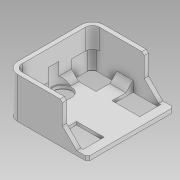
# Autodesk Inventor part: StandardPillarCover
Saved by Autodesk Inventor 2021 (Build 250183000, 183)
## iProperties
Created: 2021-03-17
Part Number: StandardPillarCover
Material: 一般
Document SubType Name: Modeling
Designer: kumagai
Density: 1 g/cm^3
Appearance: 既定
Author: kumagai
Autodesk Inventor part; units mm, degrees
ref_plane "YZ Plane" through (0, 0, 0) normal (1, 0, 0) x (0, 1, 0)
ref_plane "XZ Plane" through (0, 0, 0) normal (0, 1, 0) x (-1, 0, 0)
ref_plane "XY Plane" through (0, 0, 0) normal (0, 0, 1) x (1, 0, 0)
sketch "スケッチ1" plane through (0, 0, 0) normal (0, 1, 0) x (-1, 0, 0)
  line L0 (0, -22.1598) -> (0, 22.1598) projected
  line L1 (-9.6657, 0) -> (57.9941, 0) projected
  line L2 (43.5, -15) -> (19.2, -15)
  line L3 (19.2, -15) -> (19.2, 15)
  line L4 (19.2, 15) -> (43.5, 15)
  line L5 (47.5, 11) -> (47.5, -11)
  arc A0 (43.5, -15) -> (47.5, -11) centre (43.5, -11) ccw
  arc A1 (47.5, 11) -> (43.5, 15) centre (43.5, 11) ccw
  line L6 (44.65, -13.5) -> (37.45, -13.5)
  line L7 (37.45, -13.5) -> (37.45, -6.2)
  line L8 (37.45, -6.2) -> (46.15, -6.2)
  line L9 (46.15, -6.2) -> (46.15, -12)
  line L10 (31.85, -13.5) -> (22.25, -13.5)
  line L11 (22.25, -13.5) -> (22.25, -6.2)
  line L12 (22.25, -6.2) -> (31.85, -6.2)
  line L13 (31.85, -6.2) -> (31.85, -13.5)
  line L14 (22.25, 6.2) -> (31.85, 6.2)
  line L15 (31.85, 6.2) -> (31.85, 13.5)
  line L16 (31.85, 13.5) -> (22.25, 13.5)
  line L17 (22.25, 13.5) -> (22.25, 6.2)
  line L18 (37.45, 6.2) -> (46.15, 6.2)
  line L19 (46.15, 6.2) -> (46.15, 12)
  line L20 (44.65, 13.5) -> (37.45, 13.5)
  line L21 (37.45, 13.5) -> (37.45, 6.2)
  arc A2 (44.65, -13.5) -> (46.15, -12) centre (44.65, -12) ccw
  arc A3 (46.15, 12) -> (44.65, 13.5) centre (44.65, 12) ccw
  line L22 (28, -13.5) -> (43.5, -13.5)
  line L23 (46, -11) -> (46, 11)
  line L24 (43.5, 13.5) -> (28, 13.5)
  arc A4 (43.5, -13.5) -> (46, -11) centre (43.5, -11) ccw
  arc A5 (46, 11) -> (43.5, 13.5) centre (43.5, 11) ccw
  circle A6 centre (43, 0) radius 3.2
  line L25 (28, -13.5) -> (28, -15)
  line L26 (28, 13.5) -> (28, 15)
  point P0 (0, 0)
  point P1 (46.15, 13.5)
  dimension "d1" = 30
  dimension "d2" = 47.5
  dimension "d3" = 19.2
  dimension "d4" = 46.15
  dimension "d5" = 31.85
  dimension "d6" = 8.7
  dimension "d8" = 27
  dimension "d9" = 7.3
  dimension "d10" = 9.6
  dimension "d11" = 4
  dimension "d13" = 1.5
  dimension "d17" = 43
  dimension "d18" = 6.4
  dimension "d31" = 28
  dimension "d32" = 1.5
  constraints: 50 end point, 13 point on line, 12 point on circle, 12 tangent, 11 parallel, 9 perpendicular, 7 centre point, 5 horizontal, 2 coincident, 2 equal radius, 1 collinear, 4 other
  measures "d1" distance between parallel lines of L4 L2
  measures "d2" distance between parallel lines of L5 L0
  measures "d3" distance between parallel lines of L3 L0
  measures "d4" distance between parallel lines of L0 L9
  measures "d5" distance between parallel lines of L0 L13
  measures "d6" distance between parallel lines of L9 L7
  measures "d8" distance between parallel lines of L20 L6
  measures "d9" distance between parallel lines of L6 L8
  measures "d10" distance between parallel lines of L11 L13
  measures "d11" radius of A0
  measures "d13" radius of A2
  measures "d17" distance from line of L0 A6.centre
  measures "d18" diameter of A6
  measures "d31" distance between parallel lines of L26 L0
  measures "d32" distance between parallel lines of L2 L22
extrude "押し出し1" add sketch "スケッチ1" along normal blind 1.5 contours L3 L4 L26 L16 L17 L14 L15 L24 L21 L18 L23 A6 L1 | L1 A6 L23 L8 L7 L22 L13 L12 L11 L10 L25 L2 L3 | A6 L23 L1 | L1 L23 A6 | L23 A6 L1 | L1 A6 L23 | L23 A5 L20 A3 L19 L18 | L18 L21 L20 A5 L23 | L23 A4 L6 L7 L8 | L8 L9 A2 L6 A4 L23 | L10 L11 L12 L13 | L16 L15 L14 L17
extrude "押し出し2" add sketch "スケッチ1" along normal blind 14.2 contours L23 A6 L1 | L1 A6 L23 | L23 L18 L19 A3 L20 L24 L16 L26 L4 A1 L5 L1 A6 | A6 L1 L5 A0 L2 L25 L10 L22 L6 A2 L9 L8 L23 | L23 A5 L20 A3 L19 L18 | L8 L9 A2 L6 A4 L23 picked at (46.0369, 0.6216) picked at (46.0369, -0.6216)
chamfer "面取り1" distance 2.5 angle 45 5 edges at (-45.2678, 1.5, -12.7678) (-46, 1.5, 0) (-45.2678, 1.5, 12.7678) (-35.75, 1.5, 13.5) (-35.75, 1.5, -13.5)
extrude "押し出し3" cut sketch "スケッチ1" along normal blind 7 contours A6 L23 L1 | L1 L23 A6 | L23 A6 L1 | L1 A6 L23 | L23 A5 L20 A3 L19 L18 | L18 L21 L20 A5 L23 | L23 A4 L6 L7 L8 | L8 L9 A2 L6 A4 L23 | L10 L11 L12 L13 | L16 L15 L14 L17
sketch "スケッチ2" plane through (0, 1.5, 0) normal (0, 1, 0) x (1, 0, 0)
  arc A0 (-43.5, -3.1607) -> (-43.5, 3.1607) centre (-43, 0) ccw projected
  circle A1 centre (-43, 0) radius 3.5
  point P0 (0, 0)
  dimension "d28" = 7
  constraints: 1 centre point, 1 coincident
  measures "d28" diameter of A1
extrude "押し出し4" cut sketch "スケッチ2" along normal blind 7
chamfer "面取り2" distance 5 angle 45 2 edges at (-28, 1.5, -14.25) (-28, 1.5, 14.25)
chamfer "面取り3" distance 0.8 angle 45 4 edges at (-28, 14.2, 14.25) (-28, 14.2, -14.25) (-19.2, 0.75, -15) (-19.2, 0.75, 15)
chamfer "面取り4" distance 0.4 angle 45 19 edges at (-27.05, 0, 6.2) (-22.25, 0, 9.85) (-27.05, 0, 13.5) (-31.85, 0, 9.85) (-37.45, 0, 9.85) (-41.05, 0, 13.5) (-45.7107, 0, 13.0607) (-46.15, 0, 9.1) (-41.8, 0, 6.2) (-41.8, 0, -6.2) (-37.45, 0, -9.85) (-46.15, 0, -9.1) (-45.7107, 0, -13.0607) (-41.05, 0, -13.5) (-31.85, 0, -9.85) (-27.05, 0, -6.2) (-22.25, 0, -9.85) (-27.05, 0, -13.5) (-39.8, 0, 0)
equation "\"cp\" = 0.15"
